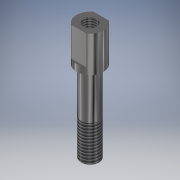
# Autodesk Inventor part: BallTransferUnit
Saved by Autodesk Inventor 2019 (Build 230136000, 136)
## iProperties
Created: 2021-03-21
Part Number: BallTransferUnit
Material: Stainless Steel
Document SubType Name: Modeling
Designer: rtavi
Density: 8 g/cm^3
Appearance: Semi-Polished
Mass: 37.498 g
Surface Area: 23.3734 cm^2
Volume: 4.68726 cm^3
Author: rtavi
Autodesk Inventor part; units mm, degrees
ref_plane "YZ Plane" through (0, 0, 0) normal (1, 0, 0) x (0, 1, 0)
ref_plane "XZ Plane" through (0, 0, 0) normal (0, 1, 0) x (-1, 0, 0)
ref_plane "XY Plane" through (0, 0, 0) normal (0, 0, 1) x (1, 0, 0)
sketch "Sketch1" plane through (0, 0, 0) normal (0, 1, 0) x (-1, 0, 0)
  arc A0 (3.3166, 5) -> (-3.3166, -5) centre (0, 0) ccw
  line L0 (3.3166, 5) -> (-3.3166, 5) construction
  line L1 (3.3166, -5) -> (-3.3166, -5) construction
  arc A1 (3.3166, 5) -> (-3.3166, 5) centre (0, 0) ccw construction
  arc A2 (3.3166, -5) -> (3.3166, 5) centre (0, 0) ccw
  arc A3 (-3.3166, -5) -> (3.3166, -5) centre (0, 0) ccw
  line L2 (0, 0) -> (18.76, 0) construction
  point P0 (5.7735, 0)
  dimension "d17" = 10
  dimension "d18" = 12
  constraints: 10 point on circle, 6 end point, 4 centre point, 3 horizontal, 2 coincident, 1 parallel, 1 point on line
  measures "d17" distance between parallel lines of L1 L0
  measures "d18" diameter of A0
extrude "Extrusion1" add sketch "Sketch1" along normal blind 16
sketch "Sketch2" plane through (0, 0, 0) normal (0, 1, 0) x (-1, 0, 0)
  circle A0 centre (0, 0) radius 4
  dimension "d3" = 8
  constraints: 1 centre point, 1 coincident
  measures "d3" diameter of A0
extrude "Extrusion2" add sketch "Sketch2" against normal blind 36
thread "Thread1" size "M8x1.25" class "6g" standard "ANSI Metric M Profile" length 16
sketch "Sketch4" plane through (0, 16, 0) normal (0, 1, 0) x (1, 0, 0)
  circle A0 centre (0, 0) radius 6 construction
  line L0 (-3.3166, -5) -> (3.3166, -5)
  line L1 (3.3166, 5) -> (-3.3166, 5)
  arc A1 (-3.3166, -5) -> (3.3166, -5) centre (0, 0) ccw
  arc A2 (3.3166, 5) -> (-3.3166, 5) centre (0, 0) ccw
  dimension "d20" = 10
  constraints: 8 point on circle, 4 end point, 2 centre point, 2 concentric, 2 parallel, 1 horizontal
  measures "d20" distance between parallel lines of L1 L0
extrude "Extrusion3" cut sketch "Sketch4" against normal blind 13
sketch "Sketch3" plane through (0, 16, 0) normal (0, 1, 0) x (1, 0, 0)
  point P0 (0, 0)
  point P1 (0, 0)
  constraints: 1 coincident
hole "Hole1" at (0, 16, 0) direction (0, -1, 0) diameter 6 depth 12
thread "Thread2" size "M6x1" class "6H" standard "ANSI Metric M Profile" full length
body "Solid1"
